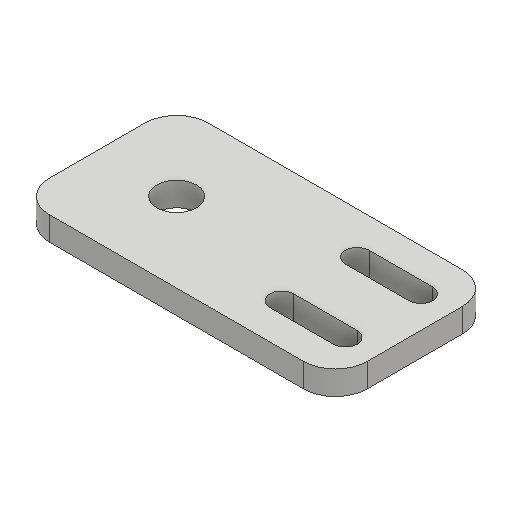
# Autodesk Inventor part: 3DP_ABS_Y_Axis_Endstop_Mount
Saved by Autodesk Inventor 2026.1 (Build 301233000, 233)
## iProperties
Created: 2017-05-25
Part Number: 3DP_ABS_Y_Axis_Endstop_Mount
Material: Ogólny
Document SubType Name: Modeling
Designer: Andrzej
Density: 1 g/cm^3
Appearance: Domyślna
Mass: 2.11348 g
Surface Area: 19.4806 cm^2
Volume: 2.11348 cm^3
Author: Andrzej
Autodesk Inventor part; units mm, degrees
ref_plane "YZ Plane" through (0, 0, 0) normal (1, 0, 0) x (0, 1, 0)
ref_plane "XZ Plane" through (0, 0, 0) normal (0, 1, 0) x (-1, 0, 0)
ref_plane "XY Plane" through (0, 0, 0) normal (0, 0, 1) x (1, 0, 0)
sketch "Szkic1" plane through (0, 0, 0) normal (0, 0, 1) x (1, 0, 0)
  line L0 (-10.9535, 6.2441) -> (21.0465, 6.2441)
  line L1 (25.0465, 2.2441) -> (25.0465, -9.7559)
  line L2 (21.0465, -13.7559) -> (-10.9535, -13.7559)
  line L3 (-14.9535, -9.7559) -> (-14.9535, 2.2441)
  arc A0 (-10.9535, 6.2441) -> (-14.9535, 2.2441) centre (-10.9535, 2.2441) ccw
  arc A1 (-14.9535, -9.7559) -> (-10.9535, -13.7559) centre (-10.9535, -9.7559) ccw
  arc A2 (21.0465, -13.7559) -> (25.0465, -9.7559) centre (21.0465, -9.7559) ccw
  arc A3 (25.0465, 2.2441) -> (21.0465, 6.2441) centre (21.0465, 2.2441) ccw
  line L4 (13.0465, 0.9941) -> (21.0465, 0.9941) construction
  line L5 (13.0465, -0.5059) -> (21.0465, -0.5059)
  line L6 (21.0465, 2.4941) -> (13.0465, 2.4941)
  arc A4 (13.0465, 2.4941) -> (13.0465, -0.5059) centre (13.0465, 0.9941) ccw
  arc A5 (21.0465, -0.5059) -> (21.0465, 2.4941) centre (21.0465, 0.9941) ccw
  line L7 (13.0465, -8.5059) -> (21.0465, -8.5059) construction
  line L8 (13.0465, -10.0059) -> (21.0465, -10.0059)
  line L9 (21.0465, -7.0059) -> (13.0465, -7.0059)
  arc A6 (13.0465, -7.0059) -> (13.0465, -10.0059) centre (13.0465, -8.5059) ccw
  arc A7 (21.0465, -10.0059) -> (21.0465, -7.0059) centre (21.0465, -8.5059) ccw
  circle A8 centre (-4.9535, -3.7559) radius 2.5
  point P0 (0, 0)
  point P1 (25.0465, -13.7559)
  point P2 (25.0465, 6.2441)
  point P3 (-14.9535, -13.7559)
  point P4 (17.0465, 0.9941)
  point P5 (17.0465, -8.5059)
  dimension "d0" = 40
  dimension "d1" = 20
  dimension "d2" = 4
  dimension "d3" = 10
  dimension "d4" = 10
  dimension "d5" = 5.25
  dimension "d6" = 5.25
  dimension "d7" = 8
  dimension "d8" = 8
  dimension "d9" = 4
  dimension "d10" = 3
  dimension "d11" = 4
  dimension "d12" = 3
  dimension "d13" = 5
  constraints: 24 end point, 16 point on circle, 16 tangent, 9 centre point, 6 point on line, 5 parallel, 3 equal radius, 2 horizontal, 2 midpoint, 1 coincident, 1 perpendicular
  measures "d0" distance of point (25.047, -13.756) point (-14.953, -13.756)
  measures "d1" distance of point (25.047, 6.244) point (25.047, -13.756)
  measures "d2" radius of A0
  measures "d3" distance from line of point (-4.953, -3.756) L3
  measures "d4" distance from line of L0 point (-4.953, -3.756)
  measures "d5" distance from line of L0 point (17.047, 0.994)
  measures "d6" distance from line of L2 point (17.047, -8.506)
  measures "d7" distance from line of L1 point (17.047, 0.994)
  measures "d8" distance from line of L1 point (17.047, -8.506)
  measures "d9" distance of point (17.047, 0.994) L4.end
  measures "d10" diameter of A5
  measures "d11" distance of point (17.047, -8.506) L7.end
  measures "d12" diameter of A7
  measures "d13" diameter of A8
extrude "Wyciągnięcie proste1" add sketch "Szkic1" along normal blind 3
equation "\"d6\" = d5"
equation "\"d8\" = d7"
